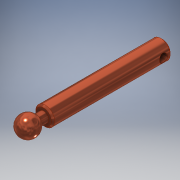
# Autodesk Inventor part: Ball_2
Saved by Autodesk Inventor 2018.1 (Build 221151000, 151)
## iProperties
Created: 2012-05-30
Part Number: Ball_2
Material: Generic
Document SubType Name: Modeling
Designer: normanpa
Density: 1 g/cm^3
Appearance: Metal 1400F Hot
Author: normanpa
Autodesk Inventor part; units mm, degrees
ref_plane "XZ Plane" through (0, 0, 0) normal (0, 1, 0) x (-1, 0, 0)
ref_plane "XY Plane" through (0, 0, 0) normal (0, 0, 1) x (1, 0, 0)
sketch "Sketch1" plane through (0, 0, 0) normal (1, 0, 0) x (0, 1, 0)
  line L0 (-5.5499, 0) -> (-5.5499, 69.85)
  line L1 (0, 0) -> (-5.5499, 0)
  line L2 (-3.0543, 69.85) -> (-5.5499, 69.85)
  line L3 (0, 73.9634) -> (0, 0)
  line L4 (-3.0543, 73.9634) -> (-3.0543, 69.85)
  line L5 (-3.0543, 73.9634) -> (0, 73.9634)
  dimension "d1" = 73.9634
  dimension "d3" = 5.5499
  dimension "d4" = 69.85
  dimension "d6" = 4.1134
  dimension "d8" = 2.4956
  constraints: 12 end point, 1 coincident, 1 parallel, 1 perpendicular, 1 vertical
  measures "d1" distance of L3.start L1.start
  measures "d3" distance of L1.start L0.start
  measures "d4" distance of L0.start L0.end
  measures "d6" distance from line of L4.start L2
  measures "d8" distance of L2.start L0.end
revolve "Revolution1" add sketch "Sketch1" angle 360 about axis through (0, 0, 73.9634) along (0, 0, -1)
sketch "Sketch2" plane through (0, 0, 0) normal (1, 0, 0) x (0, 1, 0)
  line L0 (3.0543, 73.9634) -> (-3.0543, 73.9634) construction
  arc A0 (5.9944, 79.121) -> (-5.9944, 79.121) centre (0, 79.121) ccw
  line L1 (5.5499, 69.85) -> (-5.5499, 69.85) projected
  line L2 (5.9944, 79.121) -> (-5.9944, 79.121)
  point P0 (0, 0)
  point P1 (0, 73.9634)
  point P2 (0, 69.85)
  dimension "d12" = 11.9888
  dimension "d21" = 5.1576
  dimension "d22" = 9.271
  dimension "d23" = 6.1087
  constraints: 4 end point, 3 midpoint, 2 parallel, 2 point on circle, 2 vertical alignment, 1 centre point
  measures "d12" diameter of A0
  measures "d21" distance between parallel lines of L0 L2
  measures "d22" distance between parallel lines of L2 L1
  measures "d23" distance of L0.start L0.end
revolve "Revolution2" add sketch "Sketch2" angle 360 about axis through (0, 5.9944, 79.121) along (0, -1, 0)
chamfer "Chamfer1" distance 0.9652 angle 45 2 edges at (0, 5.5499, 69.85) (0, 5.5499, 0)
ref_plane "Work Plane1" through (5.5499, 0, 34.925) normal (1, 0, 0) x (0, 1, 0)
sketch "Sketch3" plane through (5.5499, 0, 34.925) normal (1, 0, 0) x (0, 1, 0)
  point P0 (0, -34.925)
  point P1 (0, -30.099)
  dimension "d30" = 4.826
  constraints: 1 vertical alignment
  measures "d30" distance of point (0, -30.099) point (0, -34.925)
hole "Hole1" at (5.5499, 0, 4.826) direction (-1, 0, 0) diameter 4.8006 end through all
body "Solid2"
body "Solid1"
